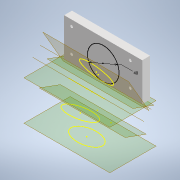
# Autodesk Inventor part: Part17
Saved by Autodesk Inventor 2021 (Build 250183000, 183)
## iProperties
Created: 2021-08-03
Part Number: Part17
Material: Generic
Document SubType Name: Modeling
Designer: Admin
Density: 1 g/cm^3
Appearance: Default
Author: Admin
Autodesk Inventor part; units mm, degrees
ref_plane "YZ Plane" through (0, 0, 0) normal (1, 0, 0) x (0, 1, 0)
ref_plane "XZ Plane" through (0, 0, 0) normal (0, 1, 0) x (-1, 0, 0)
ref_plane "XY Plane" through (0, 0, 0) normal (0, 0, 1) x (1, 0, 0)
sketch "Sketch1" plane through (0, 0, 0) normal (0, 0, 1) x (1, 0, 0)
  circle A0 centre (-40.163, 20.6) radius 1.7 projected
  circle A1 centre (34.337, 20.6) radius 1.7 projected
  circle A2 centre (-40.163, -9.9) radius 1.7 projected
  circle A3 centre (34.337, -9.9) radius 1.7 projected
  line L0 (-42.913, 23.25) -> (37.087, 23.25) projected
  line L1 (-49.577, 53) -> (-49.577, -53) construction
  line L2 (49.577, -53) -> (49.577, 53) construction
  line L3 (-49.577, 23.25) -> (49.577, 23.25)
  line L4 (-49.577, 23.25) -> (-49.577, -20)
  line L5 (49.577, 23.25) -> (49.577, -20)
  line L6 (49.577, -20) -> (-49.577, -20)
  line L7 (-47.577, -55) -> (47.577, -55) construction
  line L8 (-49.577, 23.25) -> (49.577, 23.25)
  line L9 (49.577, 23.25) -> (49.577, 28.25)
  line L10 (49.577, 28.25) -> (-49.577, 28.25)
  line L11 (-49.577, 28.25) -> (-49.577, 23.25)
  point P0 (0, 0)
  point P1 (49.577, 23.25)
  dimension "d0" = 99.154
  dimension "d2" = 5
  dimension "d3" = 10.1
  constraints: 16 end point, 6 point on line, 2 parallel, 2 perpendicular, 1 horizontal
  measures "d0" distance of L3.start L3.end
  measures "d2" distance between parallel lines of L10 L8
  measures "d3" distance from line of A2.centre L6
extrude "Extrusion1" add sketch "Sketch1" along normal blind 10
ref_plane "Work Plane1" through (-49.577, -20, 10) normal (0, -0.5, 0.8660254) x (1, 0, 0)
ref_plane "Work Plane3" through (-49.577, -29.0156, 19.0156) normal (0, -0.7071068, 0.7071068) x (1, 0, 0)
ref_plane "Work Plane2" through (-49.577, -20, 10) normal (0, -0.7071068, 0.7071068) x (1, 0, 0)
ref_plane "Work Plane5" through (-49.577, -47.0162, 19.8331) normal (0, -0.9396926, 0.3420201) x (1, 0, 0)
ref_plane "Work Plane4" through (-49.577, -20, 10) normal (0, -0.9396926, 0.3420201) x (1, 0, 0)
sketch "Sketch2" plane through (0, 0, 10) normal (0, 0, 1) x (1, 0, 0)
  circle A0 centre (0, 0) radius 20
  dimension "d11" = 40
  constraints: 1 centre point, 1 coincident
  measures "d11" diameter of A0
sketch "Sketch3" plane through (-49.577, -20, 10) normal (0, -0.5, 0.8660254) x (1, 0, 0)
  ellipse E0 centre (49.577, 17.3205) end of major axis (69.577, 17.3205) minor radius 17.3205 projected
  point P0 (49.577, 12.3205)
sketch "Sketch4" plane through (-49.577, -29.0156, 19.0156) normal (0, -0.7071068, 0.7071068) x (1, 0, 0)
  ellipse E0 centre (49.577, 16.7303) end of major axis (69.577, 16.7303) minor radius 16.7303 projected
  point P0 (49.577, 7.0711)
sketch "Sketch5" plane through (-49.577, -47.0162, 19.8331) normal (0, -0.9396926, 0.3420201) x (1, 0, 0)
  ellipse E0 centre (49.577, 20.5512) end of major axis (69.577, 20.5512) minor radius 15.1628 projected
  point P0 (49.577, -2.5565)
ref_plane "Work Plane7" through (-49.577, -70, 10) normal (0, -1, 0) x (1, 0, 0)
ref_plane "Work Plane6" through (-49.577, -20, 10) normal (0, -1, 0) x (1, 0, 0)
sketch "Sketch6" plane through (-49.577, -70, 10) normal (0, -1, 0) x (1, 0, 0)
  ellipse E0 centre (49.577, 20.8457) end of major axis (69.577, 20.8457) minor radius 11.8301 projected
  point P0 (49.577, -10)
body "Solid1"
